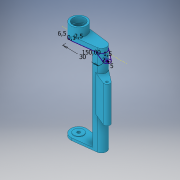
# Autodesk Inventor part: Servo-Arm-Lip
Saved by Autodesk Inventor 2018.3 (Build 223284000, 284)
## iProperties
Created: 2018-02-17
Part Number: Servo-Arm-Lip
Material: Generisch
Document SubType Name: Modeling
Designer: JochenAlt
Density: 1 g/cm^3
Appearance: Vorgabe
Author: JochenAlt
Autodesk Inventor part; units mm, degrees
ref_plane "YZ Plane" through (0, 0, 0) normal (1, 0, 0) x (0, 1, 0)
ref_plane "XZ Plane" through (0, 0, 0) normal (0, 1, 0) x (-1, 0, 0)
sketch "Skizze1" plane through (0, 0, 0) normal (0, 0, 1) x (1, 0, 0)
  line L0 (0, 5.6) -> (0, -5.6) construction
  line L1 (-9.12, 0) -> (26.72, 0) construction
  circle A0 centre (0, 0) radius 2
  circle A1 centre (9.5, 0) radius 1
  circle A2 centre (16, 0) radius 1
  circle A3 centre (19, 0) radius 1
  arc A4 (19.191579, -2.592932) -> (19.191579, 2.592932) centre (19, 0) ccw
  arc A5 (0.294737, 3.989126) -> (0.294737, -3.989126) centre (0, 0) ccw
  line L2 (0.294737, 3.989126) -> (19.191579, 2.592932)
  line L3 (0.294737, -3.989126) -> (19.191579, -2.592932)
  circle A6 centre (12.8, 0) radius 1
  circle A7 centre (0, 0) radius 4
  point P0 (0.526316, 3.965223)
  point P1 (0.657895, -1.888697)
  point P2 (0.657895, 1.888697)
  dimension "d0" = 9.5
  dimension "d1" = 16
  dimension "d2" = 19
  dimension "d3" = 5.2
  dimension "d4" = 2
  dimension "d5" = 4
  dimension "d6" = 8
  dimension "d17" = 12.8
  constraints: 7 centre point, 7 point on circle, 4 coincident, 4 end point, 4 point on line, 4 tangent, 3 equal radius, 3 other
  measures "d0" distance of A1.centre point (0, 0)
  measures "d1" distance of point (0, 0) A2.centre
  measures "d2" distance of A3.centre point (0, 0)
  measures "d3" diameter of A4
  measures "d4" diameter of A3
  measures "d5" diameter of A0
  measures "d6" diameter of A5
  measures "d17" distance of A6.centre point (0, 0)
extrude "Extrusion1" add sketch "Skizze1" along normal blind 1.8
extrude "Extrusion2" add sketch "Skizze1" against normal blind 2.7 contours A5 A7
sketch "Skizze6" plane through (0, 0, 0) normal (0, 0, 1) x (1, 0, 0)
  line L0 (0.294737, 3.989126) -> (19.191579, 2.592932) construction
  arc A0 (19.191579, -2.592932) -> (19.191579, 2.592932) centre (19, 0) ccw construction
  line L1 (19.191579, -2.592932) -> (0.294737, -3.989126) construction
  arc A1 (0.294737, -3.989126) -> (0.294737, 3.989126) centre (0, 0) ccw construction
  circle A2 centre (12.8, 0) radius 1 construction
  circle A3 centre (19, 0) radius 1 construction
  circle A4 centre (16, 0) radius 1 construction
  circle A5 centre (9.5, 0) radius 1 construction
  arc A6 (19.198947, -2.69266) -> (19.198947, 2.69266) centre (19, 0) ccw
  line L2 (19.198947, 2.69266) -> (0.302105, 4.088855)
  circle A7 centre (9.5, 0) radius 1 construction
  circle A8 centre (19, 0) radius 1
  line L3 (-14.3, 0) -> (40.3, 0) construction
  arc A9 (0.302105, 4.088855) -> (0.302105, -4.088855) centre (0, 0) ccw
  line L4 (0.302105, -4.088855) -> (19.198947, -2.69266)
  circle A10 centre (0, 0) radius 2 construction
  circle A11 centre (0, 0) radius 4.1
  circle A12 centre (0, 0) radius 1.25
  arc A13 (0.786842, 6.4522) -> (0.786842, -6.4522) centre (0, 0) ccw
  line L5 (19, 0) -> (30, -6.350853) construction
  circle A14 centre (30, -6.350853) radius 1
  circle A15 centre (30, -6.350853) radius 2.5
  arc A16 (15.990551, -2.929713) -> (15.990551, 2.929713) centre (19, 0) ccw
  line L6 (17.405712, -3.885646) -> (29.051019, -8.663738)
  line L7 (21.567924, 3.323517) -> (31.528526, -4.372569)
  line L8 (0.786842, -6.4522) -> (19.508421, -4.169114)
  arc A17 (15.990551, 2.929713) -> (15.990551, -2.929713) centre (19, 0) ccw
  line L9 (15.990551, -2.929713) -> (16.191031, -4.573667)
  line L10 (19.508421, 4.169114) -> (0.786842, 6.4522)
  line L11 (16.191031, 4.573667) -> (15.990551, 2.929713)
  dimension "d106" = 2.5
  dimension "d116" = 0.1
  dimension "d235" = 6.5
  dimension "d249" = 30
  dimension "d250" = 2
  dimension "d251" = 5
  dimension "d252" = 150
  dimension "d253" = 1.5
  constraints: 18 end point, 16 point on circle, 12 centre point, 11 coincident, 11 tangent, 4 point on line, 3 concentric, 2 perpendicular, 1 parallel
  measures "d106" diameter of A12
  measures "d116" distance between parallel lines of L4 L1
  measures "d235" radius of A13
  measures "d249" horizontal distance of L5.end point (0, 0)
  measures "d250" diameter of A14
  measures "d251" diameter of A15
  measures "d252" angle of L3 L5
  measures "d253" radial gap between concentric circles of A16 A6
extrude "Extrusion11" add sketch "Skizze6" along normal blind 2 separate body contours A6 L2 A16 L4 | L9 L8 A13 L10 L11 L2 A9 L4 | A16 L6 L8 L9 | L11 L10 A16 | A16 L8 L6
extrude "Extrusion12" add sketch "Skizze6" along normal blind 1.5 from surface at 2 contours L4 A17 L2 A6 | A6 L2 A16 L4 | L9 L8 A13 L10 L11 L2 A9 L4 | L4 A11 L2 A17 | A16 L6 L8 L9 | L11 L10 A16 | A9 A11 | A16 L8 L6 | A8 | A12 bodies 2
sketch "Skizze18" plane through (0, 0, 3.5) normal (0, 0, 1) x (0.9999808, 0.0061906, 0)
  circle A0 centre (0, 0) radius 5
  circle A1 centre (0, 0) radius 6.5
  circle A2 centre (0, 0) radius 4
  dimension "d183" = 10
  dimension "d192" = 8
  dimension "d197" = 1.5
  constraints: 3 centre point, 3 coincident
  measures "d183" diameter of A0
  measures "d192" diameter of A2
  measures "d197" radial gap between concentric circles of A1 A0
extrude "Extrusion29" add sketch "Skizze18" along normal blind 3 contours A0 | A1 bodies 2
extrude "Extrusion28" add sketch "Skizze18" along normal blind 4 from surface at 3 contours A1 bodies 2
extrude "Extrusion30" add sketch "Skizze6" along normal up to surface (3.5 mm away) contours L4 A17 L2 A6 | L4 A11 L2 A17 bodies 2
extrude "Extrusion37" add sketch "Skizze6" against normal blind 70 contours A6 L2 A16 L4 | A16 L6 L8 L9 | L11 L10 A16 | A16 L8 L6 bodies 2
extrude "Extrusion34" add sketch "Skizze6" against normal blind 2 from surface at -70 contours L4 A17 L2 A6 | A6 L2 A16 L4 | L9 L8 A13 L10 L11 L2 A9 L4 | L4 A11 L2 A17 | A16 L6 L8 L9 | L11 L10 A16 | A9 A11 | A16 L8 L6 | A8 bodies 2
extrude "Extrusion35" add sketch "Skizze6" along normal blind 0.5 from surface at -70 contours A9 A11 bodies 2
ref_plane "Arbeitsebene10" through (0, 0, -15) normal (0, 0, 1) x (1, 0, 0)
extrude "Extrusion36" add sketch "Skizze6" against normal blind 30 from surface at -15 contours A16 L8 L6 | A16 L7 A15 L6 L8 | A15 bodies 2
ref_plane "Arbeitsebene11" through (17.405712, -3.885646, -30) normal (0, 0, 1) x (0.9251538, -0.3795924, 0)
sketch "Skizze23" plane through (17.405712, -3.885646, -30) normal (0, 0, 1) x (0.9251538, -0.3795924, 0)
  line L0 (-1.672106, 0.347201) -> (-0.8626, -1.097609)
  line L1 (-14.400767, -8.682853) -> (-0.8626, -1.097609)
  arc A0 (-19.299179, 3.255702) -> (-14.400767, -8.682853) centre (-17.577923, -3.012255) ccw
  line L2 (-4.334858, 7.365083) -> (-19.299179, 3.255702)
  line L3 (-4.334858, 7.365083) -> (-3.8963, 5.768071)
  line L4 (-3.8963, 5.768071) -> (-0.838056, 6.766644)
  arc A1 (1.20617, 1.784394) -> (-0.838056, 6.766644) centre (0, 4.2) ccw
  line L5 (1.20617, 1.784394) -> (-1.672106, 0.347201)
  circle A2 centre (0, 4.2) radius 1
  circle A3 centre (-17.577923, -3.012255) radius 4.1
  line L6 (-0.838056, 6.766644) -> (-3.8963, 5.768071)
  line L7 (0.328398, 8.645669) -> (-4.334858, 7.365083)
  arc A4 (1.20617, 1.784394) -> (-0.838056, 6.766644) centre (0, 4.2) ccw
  line L8 (0.198905, 6.892664) -> (0.328398, 8.645669)
  constraints: 4 end point, 1 collinear, 1 line through centre, 1 point on circle
extrude "Extrusion40" cut sketch "Skizze23" along normal mid plane 7 contours L0 L1 A0 L2 L3 L4 A1 L5 | A1 L4 L3 L7 L8 | A2 bodies 2
fillet "Rundung9" radius 3.5 2 edges at (20.5412, 3.0866, -33.5) (20.5412, 3.0866, -26.5)
